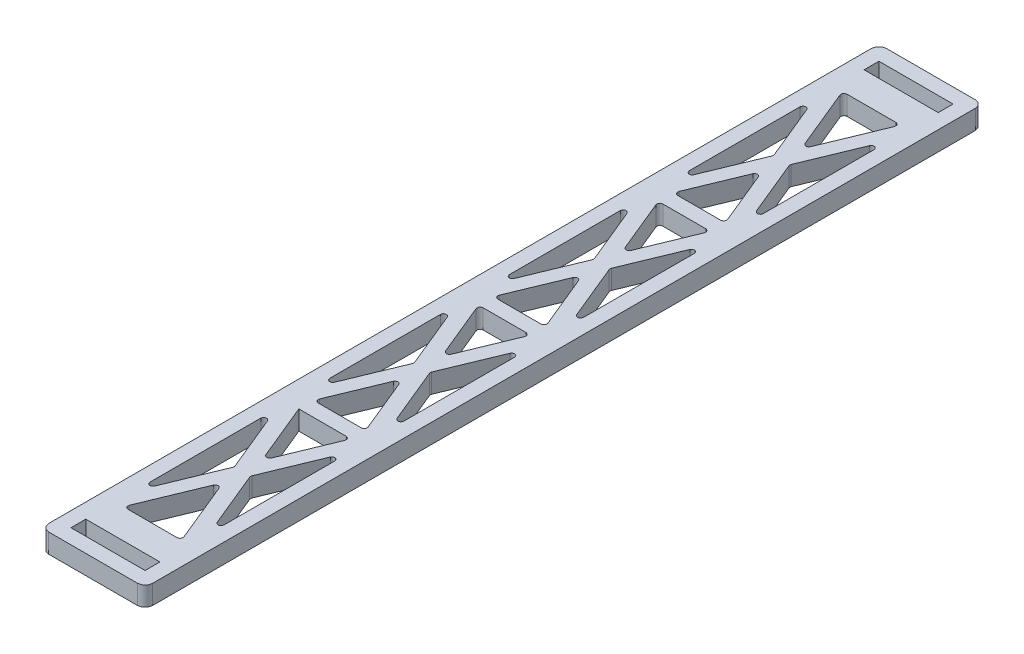
# Autodesk Inventor part: mount_battery_fastener
Saved by Autodesk Inventor 2021 (Build 250183000, 183)
## iProperties
Created: 2021-01-30
Part Number: mount_battery_fastener
Material: ABS Plastic
Document SubType Name: Modeling
Designer: User
Density: 1.06 g/cm^3
Appearance: Smooth - Black
Author: User
Autodesk Inventor part; units mm, degrees
ref_plane "YZ Plane" through (0, 0, 0) normal (1, 0, 0) x (0, 1, 0)
ref_plane "XZ Plane" through (0, 0, 0) normal (0, 1, 0) x (-1, 0, 0)
ref_plane "XY Plane" through (0, 0, 0) normal (0, 0, 1) x (1, 0, 0)
sketch "Sketch1" plane through (0, 0, 0) normal (0, 1, 0) x (-1, 0, 0)
  line L0 (-7, 0) -> (-7, 55.5)
  line L1 (-6, 56.5) -> (6, 56.5)
  line L2 (7, 55.5) -> (7, 0)
  line L3 (0, 0) -> (0, 56.5) construction
  line L4 (-5, 52.5) -> (5, 52.5)
  line L5 (5, 52.5) -> (5, 54.5)
  line L6 (5, 54.5) -> (-5, 54.5)
  line L7 (-5, 54.5) -> (-5, 52.5)
  arc A0 (-6, 56.5) -> (-7, 55.5) centre (-6, 55.5) ccw
  arc A1 (7, 55.5) -> (6, 56.5) centre (6, 55.5) ccw
  line L8 (7, 0) -> (-7, 0) construction
  line L9 (5, 48.5) -> (-5, 48.5)
  line L10 (5, 48.5) -> (5, 0)
  line L11 (-5, 48.5) -> (-5, 0)
  line L12 (5, 48.5) -> (-5, 24.25) construction
  line L13 (5, 0) -> (-5, 24.25) construction
  line L14 (-5, 0) -> (5, 24.25) construction
  line L15 (-5, 48.5) -> (5, 24.25) construction
  line L16 (-5, 24.25) -> (5, 24.25) construction
  line L17 (5, 2.6231) -> (1.0817, 12.125)
  line L18 (1.0817, 12.125) -> (5, 21.6269)
  line L19 (5, 26.8731) -> (1.0817, 36.375)
  line L20 (1.0817, 36.375) -> (5, 45.8769)
  line L21 (-1.0817, 36.375) -> (-5, 26.8731)
  line L22 (-1.0817, 36.375) -> (-5, 45.8769)
  line L23 (3.5059, 23.25) -> (0, 14.7481)
  line L24 (0, 14.7481) -> (-3.5059, 23.25)
  line L25 (-3.5059, 23.25) -> (3.5059, 23.25)
  line L26 (3.5059, 25.25) -> (-3.5059, 25.25)
  line L27 (-3.5059, 25.25) -> (0, 33.7519)
  line L28 (0, 33.7519) -> (3.5059, 25.25)
  line L29 (-1.0817, 12.125) -> (-5, 2.6231)
  line L30 (-1.0817, 12.125) -> (-5, 21.6269)
  line L31 (0, 38.9981) -> (3.9183, 48.5)
  line L32 (0, 38.9981) -> (-3.9183, 48.5)
  line L33 (3.5059, 1) -> (-3.5059, 1)
  line L34 (-3.5059, 1) -> (0, 9.5019)
  line L35 (3.5059, 1) -> (0, 9.5019)
  line L36 (-7, 0) -> (-7, -55.5)
  line L37 (-6, -56.5) -> (6, -56.5)
  line L38 (7, -55.5) -> (7, 0)
  line L39 (-5, -52.5) -> (5, -52.5)
  line L40 (5, -52.5) -> (5, -54.5)
  line L41 (5, -54.5) -> (-5, -54.5)
  line L42 (-5, -54.5) -> (-5, -52.5)
  arc A2 (-7, -55.5) -> (-6, -56.5) centre (-6, -55.5) ccw
  arc A3 (6, -56.5) -> (7, -55.5) centre (6, -55.5) ccw
  line L43 (5, -48.5) -> (-5, -48.5)
  line L44 (5, -48.5) -> (5, 0)
  line L45 (-5, -48.5) -> (-5, 0)
  line L46 (5, -48.5) -> (-5, -24.25) construction
  line L47 (5, 0) -> (-5, -24.25) construction
  line L48 (-5, 0) -> (5, -24.25) construction
  line L49 (-5, -48.5) -> (5, -24.25) construction
  line L50 (-5, -24.25) -> (5, -24.25) construction
  line L51 (5, -2.6231) -> (1.0817, -12.125)
  line L52 (1.0817, -12.125) -> (5, -21.6269)
  line L53 (5, -26.8731) -> (1.0817, -36.375)
  line L54 (1.0817, -36.375) -> (5, -45.8769)
  line L55 (-1.0817, -36.375) -> (-5, -26.8731)
  line L56 (-1.0817, -36.375) -> (-5, -45.8769)
  line L57 (3.5059, -23.25) -> (0, -14.7481)
  line L58 (0, -14.7481) -> (-3.5059, -23.25)
  line L59 (-3.5059, -23.25) -> (3.5059, -23.25)
  line L60 (3.5059, -25.25) -> (-3.5059, -25.25)
  line L61 (-3.5059, -25.25) -> (0, -33.7519)
  line L62 (0, -33.7519) -> (3.5059, -25.25)
  line L63 (-1.0817, -12.125) -> (-5, -2.6231)
  line L64 (-1.0817, -12.125) -> (-5, -21.6269)
  line L65 (0, -38.9981) -> (3.9183, -48.5)
  line L66 (0, -38.9981) -> (-3.9183, -48.5)
  line L67 (3.5059, -1) -> (-3.5059, -1)
  line L68 (-3.5059, -1) -> (0, -9.5019)
  line L69 (3.5059, -1) -> (0, -9.5019)
  point P0 (-7, 56.5)
  point P1 (7, 56.5)
  point P2 (0, 0)
  point P3 (-7, -56.5)
  point P4 (7, -56.5)
  point P5 (0, -56.5)
  dimension "d6" = 14
  dimension "d10" = 2
  dimension "d11" = 1
  dimension "d12" = 2
  dimension "d15" = 10
  dimension "d16" = 52.5
  dimension "d17" = 4
  dimension "d21" = 2
  dimension "d22" = 2
  dimension "d23" = 2
  dimension "d25" = 2
  dimension "d26" = 2
  dimension "d28" = 2
  dimension "d29" = 2
  dimension "d30" = 2
  dimension "d31" = 2
  dimension "d32" = 2
  dimension "d33" = 2
  dimension "d38" = 2
  dimension "d39" = 2
  dimension "d40" = 2
  dimension "d41" = 2
  dimension "d42" = 2
  dimension "d43" = 2
  constraints: 140 end point, 41 symmetric about line, 31 point on line, 20 parallel, 8 point on circle, 7 midpoint, 5 horizontal, 5 perpendicular, 4 centre point, 4 horizontal alignment, 4 tangent, 2 vertical alignment, 1 equal length, 1 equal radius, 1 vertical, 4 other
  measures "d6" distance of point (-7, 56.5) point (7, 56.5)
  measures "d10" distance between parallel lines of L1 L6
  measures "d11" radius of A0
  measures "d12" distance between parallel lines of L4 L6
  measures "d15" distance of L4.start L4.end
  measures "d16" distance from line of L3.start L4
  measures "d17" distance between parallel lines of L9 L4
  measures "d21" distance between parallel lines of L0 L11
  measures "d22" distance between parallel lines of L2 L10
  measures "d23" diameter of L17 L13
  measures "d25" diameter of L18 L14
  measures "d26" diameter of L23 L14
  measures "d28" diameter of L29 L14
  measures "d29" diameter of L25 L16
  measures "d30" diameter of L26 L16
  measures "d31" diameter of L28 L15
  measures "d32" diameter of L19 L15
  measures "d33" diameter of L20 L12
  measures "d38" diameter of L22 L15
  measures "d39" diameter of L21 L12
  measures "d40" diameter of L32 L15
  measures "d41" diameter of L30 L13
  measures "d42" diameter of L33 L8
  measures "d43" diameter of L35 L13
extrude "Extrusion2" add sketch "Sketch1" along normal blind 2.6 contours L0 A0 L1 A1 L2 L38 A3 L37 A2 L36 | L10 L20 L19 L18 L17 L44 L51 L52 L53 L54 L43 L65 L66 L45 L56 L55 L64 L63 L11 L29 L30 L21 L22 L9 L32 L31
fillet "Fillet1" radius 0.4 47 edges at (-5, 1.3, 45.8769) (-5, 1.3, 26.8731) (-1.0817, 1.3, 36.375) (-3.9183, 1.3, 48.5) (0, 1.3, 38.9981) (3.9183, 1.3, 48.5) (5, 1.3, 45.8769) (1.0817, 1.3, 36.375) (0, 1.3, 33.7519) (3.5059, 1.3, 25.25) (5, 1.3, 26.8731) (3.5059, 1.3, 23.25) (-3.5059, 1.3, 23.25) (-5, 1.3, 21.6269) (0, 1.3, 14.7481) (-1.0817, 1.3, 12.125) (3.5059, 1.3, 1) (-3.5059, 1.3, 1) (-5, 1.3, 2.6231) (0, 1.3, 9.5019) (1.0817, 1.3, 12.125) (5, 1.3, 2.6231) (5, 1.3, 21.6269) (-3.5059, 1.3, -1) (0, 1.3, -9.5019) (3.5059, 1.3, -1) (5, 1.3, -2.6231) (1.0817, 1.3, -12.125) (-1.0817, 1.3, -12.125) (-5, 1.3, -2.6231) (-5, 1.3, -21.6269) (-3.5059, 1.3, -23.25) (3.5059, 1.3, -23.25) (0, 1.3, -14.7481) (5, 1.3, -21.6269) (-3.5059, 1.3, -25.25) (0, 1.3, -33.7519) (3.5059, 1.3, -25.25) (5, 1.3, -26.8731) (1.0817, 1.3, -36.375) (5, 1.3, -45.8769) (3.9183, 1.3, -48.5) (-3.9183, 1.3, -48.5) (0, 1.3, -38.9981) (-5, 1.3, -45.8769) (-5, 1.3, -26.8731) (-1.0817, 1.3, -36.375)
equation "\"d21\" = link_width"
equation "\"d22\" = link_width"
equation "\"d23\" = link_width"
equation "\"d25\" = link_width"
equation "\"d26\" = link_width"
equation "\"d28\" = link_width"
equation "\"d29\" = link_width"
equation "\"d30\" = link_width"
equation "\"d31\" = link_width"
equation "\"d32\" = link_width"
equation "\"d33\" = link_width"
equation "\"d38\" = link_width"
equation "\"d39\" = link_width"
equation "\"d40\" = link_width"
equation "\"d41\" = link_width"
equation "\"d42\" = link_width"
equation "\"d43\" = link_width"
equation "\"link_width\" = 2"
body "Solid2"
